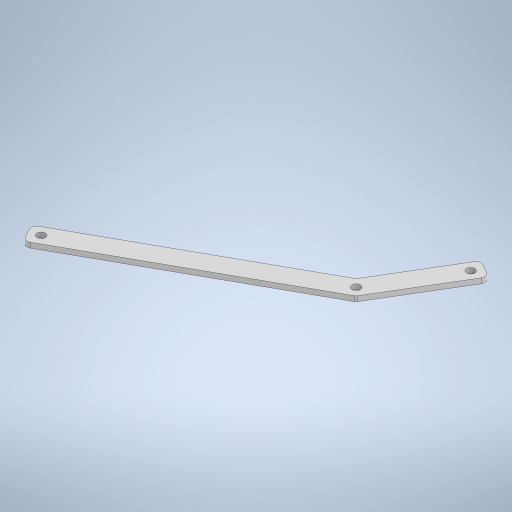
# Autodesk Inventor part: Outer Gripper Bar
Saved by Autodesk Inventor 2023 (Build 270158000, 158)
## iProperties
Created: 2023-03-01
Part Number: Outer Gripper Bar
Material: Generic
Document SubType Name: Modeling
Designer: Gabriel - T3 CAD
Density: 1 g/cm^3
Appearance: Default
Author: Gabriel - T3 CAD
Autodesk Inventor part; units mm, degrees
ref_plane "YZ Plane" through (0, 0, 0) normal (1, 0, 0) x (0, 1, 0)
ref_plane "XZ Plane" through (0, 0, 0) normal (0, 1, 0) x (-1, 0, 0)
ref_plane "XY Plane" through (0, 0, 0) normal (0, 0, 1) x (1, 0, 0)
sketch "Sketch1" plane through (0, 0, 0) normal (0, 1, 0) x (-1, 0, 0)
  line L0 (0, 76.2) -> (0, -76.2)
  line L1 (270.7338, 0) -> (-270.7338, 0)
  circle A0 centre (0, 69.85) radius 2.5797
  circle A1 centre (0, 44.45) radius 2.5797
  circle A2 centre (152.4, 158.75) radius 2.5797
  line L2 (158.75, 139.7) -> (158.75, 152.4)
  line L3 (158.75, 152.4) -> (273.05, 152.4)
  line L4 (273.05, 152.4) -> (273.05, 139.7)
  line L5 (273.05, 139.7) -> (158.75, 139.7)
  line L6 (146.05, 155.575) -> (158.75, 155.575)
  line L7 (158.75, 155.575) -> (158.75, 190.5)
  line L8 (158.75, 190.5) -> (146.05, 190.5)
  line L9 (146.05, 190.5) -> (146.05, 155.575)
  line L10 (158.75, 152.4) -> (273.05, 152.4)
  line L11 (273.05, 152.4) -> (273.05, 155.575)
  line L12 (273.05, 155.575) -> (158.75, 155.575)
  line L13 (158.75, 155.575) -> (158.75, 152.4)
  line L14 (158.75, 190.5) -> (273.05, 155.575)
  line L15 (266.7, 157.5153) -> (266.7, 155.575)
  circle A3 centre (152.4, 184.15) radius 2.5797
  circle A4 centre (152.4, 158.75) radius 2.5797
  line L16 (158.75, 155.575) -> (146.05, 155.575)
  line L17 (146.05, 155.575) -> (146.05, 152.4)
  line L18 (146.05, 152.4) -> (158.75, 152.4)
  line L19 (158.75, 152.4) -> (158.75, 155.575)
  line L20 (1.5875, 76.2) -> (-4.7625, 76.2)
  line L21 (-4.7625, 76.2) -> (-4.7625, -76.2)
  line L22 (-4.7625, -76.2) -> (1.5875, -76.2)
  line L23 (4.7625, -73.025) -> (4.7625, -41.275)
  line L24 (1.5875, -76.2) -> (1.5875, 76.2)
  line L25 (-1.5875, -76.2) -> (-1.5875, 76.2)
  circle A5 centre (0, -44.45) radius 2.5797
  circle A6 centre (0, -69.85) radius 2.5797
  line L26 (-4.7625, -38.1) -> (1.5875, -38.1)
  arc A7 (4.7625, -41.275) -> (1.5875, -38.1) centre (1.5875, -41.275) ccw
  arc A8 (1.5875, -76.2) -> (4.7625, -73.025) centre (1.5875, -73.025) ccw
  line L27 (-4.7625, 76.2) -> (4.7625, 76.2)
  line L28 (4.7625, 73.025) -> (4.7625, 41.275)
  line L29 (1.5875, 38.1) -> (-4.7625, 38.1)
  line L30 (-4.7625, 38.1) -> (-4.7625, 76.2)
  circle A9 centre (0, 69.85) radius 2.5797
  circle A10 centre (0, 44.45) radius 2.5797
  arc A11 (4.7625, 73.025) -> (1.5875, 76.2) centre (1.5875, 73.025) ccw
  arc A12 (1.5875, 38.1) -> (4.7625, 41.275) centre (1.5875, 41.275) ccw
  line L31 (152.4, 158.75) -> (27.7437, 90.2444)
  line L32 (27.7437, 90.2444) -> (0, 44.45)
  line L33 (5.4311, 41.1597) -> (-5.4311, 47.7403)
  line L34 (-5.4311, 47.7403) -> (22.7534, 94.2623)
  line L35 (32.6024, 100.1603) -> (38.8737, 96.361)
  line L36 (31.8523, 84.7712) -> (5.4311, 41.1597)
  line L37 (149.3417, 164.315) -> (155.4583, 153.185)
  line L38 (155.4583, 153.185) -> (33.0387, 85.9086)
  line L39 (21.1631, 79.3823) -> (17.6317, 85.8082)
  line L40 (23.9398, 95.3997) -> (149.3417, 164.315)
  arc A13 (23.9398, 95.3997) -> (22.7534, 94.2623) centre (25.4689, 92.6172) ccw
  arc A14 (33.0387, 85.9086) -> (31.8523, 84.7712) centre (34.5678, 83.1261) ccw
  circle A15 centre (152.4, 158.75) radius 2.5797
  circle A16 centre (0, 44.45) radius 2.5797
  line L41 (-5.4311, 47.7403) -> (5.4311, 41.1597)
  line L42 (5.4311, 41.1597) -> (3.7859, 38.4442)
  line L43 (-0.5748, 37.3738) -> (-6.0058, 40.6641)
  line L44 (-7.0762, 45.0248) -> (-5.4311, 47.7403)
  arc A17 (-7.0762, 45.0248) -> (-6.0058, 40.6641) centre (-4.3607, 43.3796) ccw
  arc A18 (-0.5748, 37.3738) -> (3.7859, 38.4442) centre (1.0704, 40.0893) ccw
  line L45 (149.3417, 164.315) -> (155.4583, 153.185)
  line L46 (155.4583, 153.185) -> (158.2408, 154.7141)
  line L47 (159.4942, 159.0258) -> (156.4359, 164.5908)
  line L48 (152.1242, 165.8442) -> (149.3417, 164.315)
  arc A19 (156.4359, 164.5908) -> (152.1242, 165.8442) centre (153.6534, 163.0616) ccw
  arc A20 (158.2408, 154.7141) -> (159.4942, 159.0258) centre (156.7116, 157.4966) ccw
  line L49 (152.4, 184.15) -> (26.6539, 114.3)
  line L50 (26.6539, 114.3) -> (0, 69.85)
  line L51 (5.4459, 66.5844) -> (-5.4459, 73.1156)
  line L52 (-5.4459, 73.1156) -> (21.6455, 118.2952)
  line L53 (31.4676, 124.2379) -> (37.756, 120.4671)
  line L54 (30.7873, 108.8455) -> (5.4459, 66.5844)
  line L55 (149.3165, 189.7011) -> (155.4835, 178.5989)
  line L56 (155.4835, 178.5989) -> (31.9686, 109.9883)
  line L57 (20.1227, 103.4081) -> (16.5622, 109.8179)
  line L58 (22.8267, 119.438) -> (149.3165, 189.7011)
  arc A21 (22.8267, 119.438) -> (21.6455, 118.2952) centre (24.3684, 116.6624) ccw
  arc A22 (31.9686, 109.9883) -> (30.7873, 108.8455) centre (33.5103, 107.2127) ccw
  circle A23 centre (152.4, 184.15) radius 2.5797
  circle A24 centre (26.6539, 114.3) radius 2.5797
  circle A25 centre (0, 69.85) radius 2.5797
  line L59 (-5.4459, 73.1156) -> (5.4459, 66.5844)
  line L60 (5.4459, 66.5844) -> (3.8132, 63.8614)
  line L61 (-0.5426, 62.7713) -> (-5.9886, 66.0368)
  line L62 (-7.0787, 70.3926) -> (-5.4459, 73.1156)
  arc A26 (-7.0787, 70.3926) -> (-5.9886, 66.0368) centre (-4.3558, 68.7598) ccw
  arc A27 (-0.5426, 62.7713) -> (3.8132, 63.8614) centre (1.0902, 65.4942) ccw
  line L63 (149.3165, 189.7011) -> (155.4835, 178.5989)
  line L64 (155.4835, 178.5989) -> (158.2591, 180.1407)
  line L65 (159.4928, 184.458) -> (156.4093, 190.0091)
  line L66 (152.092, 191.2428) -> (149.3165, 189.7011)
  arc A28 (156.4093, 190.0091) -> (152.092, 191.2428) centre (153.6338, 188.4673) ccw
  arc A29 (158.2591, 180.1407) -> (159.4928, 184.458) centre (156.7173, 182.9162) ccw
  line L67 (33.0039, 28.575) -> (33.0039, -28.575)
  line L68 (29.8289, -31.75) -> (23.4789, -31.75)
  line L69 (20.3039, -28.575) -> (20.3039, 28.575)
  line L70 (23.4789, 31.75) -> (29.8289, 31.75)
  line L71 (33.0039, 117.475) -> (33.0039, 22.225)
  line L72 (29.8289, 19.05) -> (23.4789, 19.05)
  line L73 (20.3039, 22.225) -> (20.3039, 117.475)
  line L74 (23.4789, 120.65) -> (29.8289, 120.65)
  circle A30 centre (26.6539, 25.4) radius 2.6206
  circle A31 centre (26.6539, -25.4) radius 2.6206
  circle A32 centre (26.6539, 25.4) radius 2.6206
  circle A33 centre (26.6539, 114.3) radius 2.6206
  arc A34 (33.0039, 28.575) -> (29.8289, 31.75) centre (29.8289, 28.575) ccw
  arc A35 (23.4789, 31.75) -> (20.3039, 28.575) centre (23.4789, 28.575) ccw
  arc A36 (20.3039, -28.575) -> (23.4789, -31.75) centre (23.4789, -28.575) ccw
  arc A37 (29.8289, -31.75) -> (33.0039, -28.575) centre (29.8289, -28.575) ccw
  arc A38 (20.3039, 22.225) -> (23.4789, 19.05) centre (23.4789, 22.225) ccw
  arc A39 (29.8289, 19.05) -> (33.0039, 22.225) centre (29.8289, 22.225) ccw
  arc A40 (33.0039, 117.475) -> (29.8289, 120.65) centre (29.8289, 117.475) ccw
  arc A41 (23.4789, 120.65) -> (20.3039, 117.475) centre (23.4789, 117.475) ccw
  point P0 (0, 0)
  point P1 (0, 0)
  point P2 (0, 44.45)
  point P3 (46.8631, 0)
  point P4 (2.1408, 35.7286)
  point P5 (161.0233, 156.2433)
  point P6 (2.1804, 61.1385)
  point P7 (161.0346, 181.6825)
  point P8 (33.0039, 31.75)
  point P9 (33.0039, -31.75)
  point P10 (33.0039, 120.65)
  point P11 (33.0039, 19.05)
  point P12 (20.3039, 19.05)
  point P13 (33.0039, 0)
  dimension "d4" = 5.1594
  dimension "d11" = 5.1594
  dimension "d17" = 152.4
  dimension "d56" = 12.7
  dimension "d57" = 114.3
  dimension "d58" = 3.175
  dimension "d61" = 6.35
  dimension "d63" = 5.1594
  dimension "d65" = 6.35
  dimension "d66" = 6.35
  dimension "d67" = 6.35
  dimension "d68" = 6.35
  dimension "d69" = 9.525
  dimension "d70" = 152.4
  dimension "d71" = 3.175
  dimension "d72" = 3.175
  dimension "d73" = 25.4
  dimension "d74" = 6.35
  dimension "d75" = 4.7625
  dimension "d76" = 4.7625
  dimension "d77" = 6.35
  dimension "d78" = 3.175
  dimension "d79" = 5.1594
  dimension "d80" = 25.4
  dimension "d81" = 6.35
  dimension "d82" = 4.7625
  dimension "d83" = 4.7625
  dimension "d84" = 6.35
  dimension "d85" = 3.175
  dimension "d89" = 190.5
  dimension "d92" = 150
  dimension "d94" = 142.24
  dimension "d95" = 12.7
  dimension "d96" = 3.175
  dimension "d97" = 6.35
  dimension "d98" = 3.175
  dimension "d99" = 6.35
  dimension "d100" = 3.175
  dimension "d101" = 5.1594
  dimension "d102" = 190.5
  dimension "d103" = 150
  dimension "d105" = 12.7
  dimension "d106" = 3.175
  dimension "d107" = 6.35
  dimension "d108" = 3.175
  dimension "d109" = 6.35
  dimension "d110" = 3.175
  dimension "d111" = 5.1594
  dimension "d112" = 12.7
  dimension "d113" = 12.7
  dimension "d114" = 76.2
  dimension "d115" = 4.7625
  dimension "d116" = 265.9713
  dimension "d117" = 42.1006
  dimension "d118" = 139.7
  dimension "d119" = 88.9
  dimension "d120" = 25.4
  dimension "d121" = 12.7
  dimension "d123" = 12.7
  dimension "d124" = 5.2413
  dimension "d125" = 6.35
  dimension "d126" = 6.35
  dimension "d127" = 6.35
  dimension "d128" = 6.35
  constraints: 150 end point, 49 tangent, 48 point on circle, 42 centre point, 42 point on line, 38 parallel, 24 equal radius, 18 perpendicular, 13 midpoint, 12 coincident, 5 vertical, 4 collinear, 1 concentric, 1 horizontal
  measures "d4" diameter of A0
  measures "d11" diameter of A1
  measures "d17" distance of L0.start L0.end
  measures "d56" distance of L2.start L2.end
  measures "d57" distance of L4.end L2.start
  measures "d58" distance of L11.end L3.end
  measures "d61" distance of L15.end L11.end
  measures "d63" diameter of A4
  measures "d65" distance from line of L9 A4.centre
  measures "d66" distance from line of L9 A3.centre
  measures "d67" distance from line of L8 A3.centre
  measures "d68" distance from line of L18 A4.centre
  measures "d69" distance of L27.end L20.end
  measures "d70" distance of L20.end L21.end
  measures "d71" distance between parallel lines of L23 L24
  measures "d72" distance between parallel lines of L21 L25
  measures "d73" distance of A6.centre A5.centre
  measures "d74" distance from line of L22 A6.centre
  measures "d75" distance from line of L21 A6.centre
  measures "d76" distance from line of L21 A5.centre
  measures "d77" distance from line of A5.centre L26
  measures "d78" radius of A7
  measures "d79" diameter of A6
  measures "d80" distance of A10.centre A9.centre
  measures "d81" distance from line of L20 A9.centre
  measures "d82" distance from line of L21 A9.centre
  measures "d83" distance from line of L21 A10.centre
  measures "d84" distance from line of L29 A10.centre
  measures "d85" radius of A11
  measures "d89" distance of L31.start L32.end
  measures "d92" angle of L31 L32
  measures "d94" distance of L31.start L31.end
  measures "d95" distance of L33.start L33.end
  measures "d96" radius of A13
  measures "d97" distance of L33.start point (2.141, 35.729)
  measures "d98" radius of A17
  measures "d99" distance of point (161.023, 156.243) L37.end
  measures "d100" radius of A19
  measures "d101" diameter of A15
  measures "d102" distance of L49.start L50.end
  measures "d103" angle of L49 L50
  measures "d105" distance of L54.end L52.start
  measures "d106" radius of A21
  measures "d107" distance of L54.end point (2.18, 61.138)
  measures "d108" radius of A26
  measures "d109" distance of point (161.035, 181.682) L64.start
  measures "d110" radius of A28
  measures "d111" diameter of A23
  measures "d112" distance between parallel lines of L38 L40
  measures "d113" distance between parallel lines of L56 L58
  measures "d114" diameter of L26 L1
  measures "d115" distance between parallel lines of L0 L23
  measures "d116" distance from line of L1.start L23
  measures "d117" distance from line of point (46.863, 0) L23
  measures "d118" diameter of point (0, 69.85) L1
  measures "d119" diameter of point (0, 44.45) L1
  measures "d120" distance of A4.centre A3.centre
  measures "d121" distance of L7.end L8.end
  measures "d123" distance of point (33.004, 19.05) point (20.304, 19.05)
  measures "d124" diameter of A31
  measures "d125" distance from line of L69 A31.centre
  measures "d126" distance from line of L69 A30.centre
  measures "d127" distance from line of L73 A32.centre
  measures "d128" distance from line of L73 A33.centre
sketch "Sketch2" plane through (0, 0, 0) normal (1, 0, 0) x (0, 1, 0)
  line L0 (0, 76.2) -> (0, -76.2)
  line L1 (270.7338, 0) -> (-270.7338, 0)
  circle A0 centre (0, 69.85) radius 2.5797
  circle A1 centre (0, 44.45) radius 2.5797
  circle A2 centre (188.7991, 19.05) radius 2.5797
  line L2 (195.1491, 0) -> (195.1491, 12.7)
  line L3 (195.1491, 12.7) -> (309.4491, 12.7)
  line L4 (309.4491, 12.7) -> (309.4491, 0)
  line L5 (309.4491, 0) -> (195.1491, 0)
  line L6 (182.4491, 15.875) -> (195.1491, 15.875)
  line L7 (195.1491, 15.875) -> (195.1491, 50.8)
  line L8 (195.1491, 50.8) -> (182.4491, 50.8)
  line L9 (182.4491, 50.8) -> (182.4491, 15.875)
  line L10 (195.1491, 12.7) -> (309.4491, 12.7)
  line L11 (309.4491, 12.7) -> (309.4491, 15.875)
  line L12 (309.4491, 15.875) -> (195.1491, 15.875)
  line L13 (195.1491, 15.875) -> (195.1491, 12.7)
  line L14 (195.1491, 50.8) -> (309.4491, 15.875)
  line L15 (303.0991, 17.8153) -> (303.0991, 15.875)
  circle A3 centre (188.7991, 44.45) radius 2.5797
  circle A4 centre (188.7991, 19.05) radius 2.5797
  line L16 (195.1491, 15.875) -> (182.4491, 15.875)
  line L17 (182.4491, 15.875) -> (182.4491, 12.7)
  line L18 (182.4491, 12.7) -> (195.1491, 12.7)
  line L19 (195.1491, 12.7) -> (195.1491, 15.875)
  line L20 (1.5875, 76.2) -> (-4.7625, 76.2)
  line L21 (-4.7625, 76.2) -> (-4.7625, -76.2)
  line L22 (-4.7625, -76.2) -> (1.5875, -76.2)
  line L23 (4.7625, -73.025) -> (4.7625, -41.275)
  line L24 (1.5875, -76.2) -> (1.5875, 76.2)
  line L25 (-1.5875, -76.2) -> (-1.5875, 76.2)
  circle A5 centre (0, -44.45) radius 2.5797
  circle A6 centre (0, -69.85) radius 2.5797
  line L26 (-4.7625, -38.1) -> (1.5875, -38.1)
  arc A7 (4.7625, -41.275) -> (1.5875, -38.1) centre (1.5875, -41.275) ccw
  arc A8 (1.5875, -76.2) -> (4.7625, -73.025) centre (1.5875, -73.025) ccw
  line L27 (-4.7625, 76.2) -> (4.7625, 76.2)
  line L28 (4.7625, 73.025) -> (4.7625, 41.275)
  line L29 (1.5875, 38.1) -> (-4.7625, 38.1)
  line L30 (-4.7625, 38.1) -> (-4.7625, 76.2)
  circle A9 centre (0, 69.85) radius 2.5797
  circle A10 centre (0, 44.45) radius 2.5797
  arc A11 (4.7625, 73.025) -> (1.5875, 76.2) centre (1.5875, 73.025) ccw
  arc A12 (1.5875, 38.1) -> (4.7625, 41.275) centre (1.5875, 41.275) ccw
  line L31 (188.7991, 19.05) -> (51.8933, 57.638)
  line L32 (51.8933, 57.638) -> (0, 44.45)
  line L33 (1.564, 38.2956) -> (-1.564, 50.6044)
  line L34 (-1.564, 50.6044) -> (51.1538, 64.0019)
  line L35 (62.311, 61.2991) -> (64.117, 54.1926)
  line L36 (50.9838, 50.855) -> (1.564, 38.2956)
  line L37 (190.5218, 25.1619) -> (187.0764, 12.9381)
  line L38 (187.0764, 12.9381) -> (52.6271, 50.8337)
  line L39 (39.5846, 54.5099) -> (41.5738, 61.5673)
  line L40 (52.7972, 63.9806) -> (190.5218, 25.1619)
  arc A13 (52.7972, 63.9806) -> (51.1538, 64.0019) centre (51.9358, 60.9247) ccw
  arc A14 (52.6271, 50.8337) -> (50.9838, 50.855) centre (51.7658, 47.7778) ccw
  circle A15 centre (188.7991, 19.05) radius 2.5797
  circle A16 centre (0, 44.45) radius 2.5797
  line L41 (-1.564, 50.6044) -> (1.564, 38.2956)
  line L42 (1.564, 38.2956) -> (-1.5131, 37.5136)
  line L43 (-5.3723, 39.8088) -> (-6.9364, 45.9631)
  line L44 (-4.6412, 49.8223) -> (-1.564, 50.6044)
  arc A17 (-4.6412, 49.8223) -> (-6.9364, 45.9631) centre (-3.8592, 46.7452) ccw
  arc A18 (-5.3723, 39.8088) -> (-1.5131, 37.5136) centre (-2.2952, 40.5908) ccw
  line L45 (190.5218, 25.1619) -> (187.0764, 12.9381)
  line L46 (187.0764, 12.9381) -> (190.1323, 12.0768)
  line L47 (194.0496, 14.2714) -> (195.7723, 20.3833)
  line L48 (193.5777, 24.3005) -> (190.5218, 25.1619)
  arc A19 (195.7723, 20.3833) -> (193.5777, 24.3005) centre (192.7163, 21.2446) ccw
  arc A20 (190.1323, 12.0768) -> (194.0496, 14.2714) centre (190.9937, 15.1327) ccw
  line L49 (194.0712, 39.6953) -> (195.7661, 45.8149)
  arc A21 (190.164, 37.4829) -> (194.0712, 39.6953) centre (191.0114, 40.5427) ccw
  arc A22 (195.7661, 45.8149) -> (193.5538, 49.7222) centre (192.7063, 46.6624) ccw
  line L50 (187.1042, 38.3304) -> (190.164, 37.4829)
  line L51 (193.5538, 49.7222) -> (190.494, 50.5696)
  circle A23 centre (188.7991, 44.45) radius 2.5797
  line L52 (190.494, 50.5696) -> (187.1042, 38.3304)
  line L53 (190.494, 50.5696) -> (187.1042, 38.3304)
  line L54 (60.5746, 86.5522) -> (62.4129, 79.4541)
  line L55 (187.1042, 38.3304) -> (50.9384, 76.043)
  line L56 (188.7991, 44.45) -> (50.1736, 82.8439)
  line L57 (51.0487, 89.1906) -> (190.494, 50.5696)
  line L58 (49.2949, 76.0568) -> (1.592, 63.7028)
  line L59 (-1.592, 75.9972) -> (49.4052, 89.2043)
  line L60 (50.1736, 82.8439) -> (0, 69.85)
  arc A24 (50.9384, 76.043) -> (49.2949, 76.0568) centre (50.0909, 72.9832) ccw
  arc A25 (51.0487, 89.1906) -> (49.4052, 89.2043) centre (50.2012, 86.1307) ccw
  circle A26 centre (50.1736, 82.8439) radius 2.5797
  line L61 (37.8792, 79.6599) -> (39.8363, 86.7262)
  line L62 (1.592, 63.7028) -> (-1.592, 75.9972)
  line L63 (1.592, 63.7028) -> (-1.4816, 62.9068)
  line L64 (-1.592, 75.9972) -> (1.592, 63.7028)
  circle A27 centre (0, 69.85) radius 2.5797
  line L65 (-4.6656, 75.2012) -> (-1.592, 75.9972)
  arc A28 (-5.3512, 65.1844) -> (-1.4816, 62.9068) centre (-2.2776, 65.9804) ccw
  line L66 (-5.3512, 65.1844) -> (-6.9432, 71.3316)
  arc A29 (-4.6656, 75.2012) -> (-6.9432, 71.3316) centre (-3.8696, 72.1276) ccw
  line L67 (124.3721, 28.575) -> (124.3721, -28.575)
  line L68 (121.1971, -31.75) -> (114.8471, -31.75)
  line L69 (111.6721, -28.575) -> (111.6721, 28.575)
  line L70 (114.8471, 31.75) -> (121.1971, 31.75)
  line L71 (51.8536, 89.7417) -> (124.5484, 28.1948)
  line L72 (124.92, 23.72) -> (120.8168, 18.8737)
  line L73 (116.3421, 18.5021) -> (43.6473, 80.0491)
  line L74 (43.2757, 84.5238) -> (47.3789, 89.3701)
  circle A30 centre (118.0221, 25.4) radius 2.6206
  circle A31 centre (118.0221, -25.4) radius 2.6206
  circle A32 centre (118.0221, 25.4) radius 2.6206
  circle A33 centre (50.1736, 82.8439) radius 2.6206
  arc A34 (124.3721, 28.575) -> (121.1971, 31.75) centre (121.1971, 28.575) ccw
  arc A35 (114.8471, 31.75) -> (111.6721, 28.575) centre (114.8471, 28.575) ccw
  arc A36 (111.6721, -28.575) -> (114.8471, -31.75) centre (114.8471, -28.575) ccw
  arc A37 (121.1971, -31.75) -> (124.3721, -28.575) centre (121.1971, -28.575) ccw
  arc A38 (116.3421, 18.5021) -> (120.8168, 18.8737) centre (118.3937, 20.9253) ccw
  arc A39 (124.92, 23.72) -> (124.5484, 28.1948) centre (122.4968, 25.7716) ccw
  arc A40 (51.8536, 89.7417) -> (47.3789, 89.3701) centre (49.802, 87.3186) ccw
  arc A41 (43.2757, 84.5238) -> (43.6473, 80.0491) centre (45.6989, 82.4723) ccw
  line L75 (50.1736, 82.8439) -> (118.0221, 25.4)
  line L76 (118.0221, -25.4) -> (118.0221, 25.4)
  line L77 (127.9831, -605.0736) -> (127.9831, -452.6736)
  line L78 (178.1568, -446.0297) -> (246.0052, -503.4736)
  line L79 (246.0052, -503.4736) -> (246.0052, -554.2736)
  line L80 (78.5716, -330.2354) -> (78.5716, -190.5354)
  line L81 (78.5716, -190.5354) -> (172.9711, -203.2354)
  line L82 (172.9711, -203.2354) -> (256.0081, -234.9854)
  line L83 (256.0081, -234.9854) -> (256.0081, -285.7854)
  line L84 (78.5716, -260.3854) -> (256.0081, -260.3854)
  line L85 (127.9831, -528.8736) -> (246.0052, -528.8736)
  line L86 (127.9831, -459.0236) -> (178.1568, -446.0297)
  line L87 (78.5716, -190.5354) -> (267.3706, -215.9354)
  line L88 (267.3706, -215.9354) -> (267.3706, -260.3854)
  point P0 (0, 0)
  point P1 (0, 0)
  point P2 (0, 44.45)
  point P3 (46.8631, 0)
  point P4 (-4.5903, 36.7316)
  point P5 (193.1883, 11.2155)
  point P6 (193.2238, 36.6355)
  point P7 (-4.5552, 62.1108)
  point P8 (124.3721, 31.75)
  point P9 (124.3721, -31.75)
  point P10 (49.4304, 91.7933)
  point P11 (126.9715, 26.1432)
  point P12 (118.7653, 16.4505)
  point P13 (124.3721, 0)
  point P14 (118.0221, 0)
  dimension "d145" = 5.1594
  dimension "d146" = 5.1594
  dimension "d147" = 152.4
  dimension "d148" = 12.7
  dimension "d149" = 114.3
  dimension "d150" = 3.175
  dimension "d151" = 6.35
  dimension "d152" = 5.1594
  dimension "d153" = 6.35
  dimension "d154" = 6.35
  dimension "d155" = 6.35
  dimension "d156" = 6.35
  dimension "d157" = 9.525
  dimension "d158" = 152.4
  dimension "d159" = 3.175
  dimension "d160" = 3.175
  dimension "d161" = 25.4
  dimension "d162" = 6.35
  dimension "d163" = 4.7625
  dimension "d164" = 4.7625
  dimension "d165" = 6.35
  dimension "d166" = 3.175
  dimension "d167" = 5.1594
  dimension "d168" = 25.4
  dimension "d169" = 6.35
  dimension "d170" = 4.7625
  dimension "d171" = 4.7625
  dimension "d172" = 6.35
  dimension "d173" = 3.175
  dimension "d174" = 190.5
  dimension "d175" = 150
  dimension "d176" = 142.24
  dimension "d177" = 12.7
  dimension "d178" = 3.175
  dimension "d179" = 6.35
  dimension "d180" = 3.175
  dimension "d181" = 6.35
  dimension "d182" = 3.175
  dimension "d183" = 5.1594
  dimension "d184" = 190.5
  dimension "d185" = 150
  dimension "d186" = 12.7
  dimension "d187" = 3.175
  dimension "d188" = 6.35
  dimension "d189" = 3.175
  dimension "d190" = 6.35
  dimension "d191" = 3.175
  dimension "d192" = 5.1594
  dimension "d193" = 12.7
  dimension "d194" = 12.7
  dimension "d195" = 76.2
  dimension "d196" = 4.7625
  dimension "d197" = 265.9713
  dimension "d198" = 42.1006
  dimension "d199" = 139.7
  dimension "d200" = 88.9
  dimension "d201" = 25.4
  dimension "d202" = 12.7
  dimension "d203" = 12.7
  dimension "d204" = 5.2413
  dimension "d205" = 6.35
  dimension "d206" = 6.35
  dimension "d207" = 6.35
  dimension "d208" = 6.35
  constraints: 182 end point, 49 tangent, 48 point on circle, 44 point on line, 42 centre point, 38 parallel, 24 equal radius, 19 midpoint, 18 perpendicular, 12 coincident, 8 vertical, 5 collinear, 3 horizontal, 2 equal length, 1 concentric
  measures "d145" diameter of A0
  measures "d146" diameter of A1
  measures "d147" distance of L0.start L0.end
  measures "d148" distance of L2.start L2.end
  measures "d149" distance of L4.end L2.start
  measures "d150" distance of L11.end L3.end
  measures "d151" distance of L15.end L11.end
  measures "d152" diameter of A4
  measures "d153" distance from line of L9 A4.centre
  measures "d154" distance from line of L9 A3.centre
  measures "d155" distance from line of L8 A3.centre
  measures "d156" distance from line of L18 A4.centre
  measures "d157" distance of L27.end L20.end
  measures "d158" distance of L20.end L21.end
  measures "d159" distance between parallel lines of L23 L24
  measures "d160" distance between parallel lines of L21 L25
  measures "d161" distance of A6.centre A5.centre
  measures "d162" distance from line of L22 A6.centre
  measures "d163" distance from line of L21 A6.centre
  measures "d164" distance from line of L21 A5.centre
  measures "d165" distance from line of A5.centre L26
  measures "d166" radius of A7
  measures "d167" diameter of A6
  measures "d168" distance of A10.centre A9.centre
  measures "d169" distance from line of L20 A9.centre
  measures "d170" distance from line of L21 A9.centre
  measures "d171" distance from line of L21 A10.centre
  measures "d172" distance from line of L29 A10.centre
  measures "d173" radius of A11
  measures "d174" distance of L31.start L32.end
  measures "d175" angle of L31 L32
  measures "d176" distance of L31.start L31.end
  measures "d177" distance of L33.start L33.end
  measures "d178" radius of A13
  measures "d179" distance of L33.start point (-4.59, 36.732)
  measures "d180" radius of A17
  measures "d181" distance of point (193.188, 11.215) L37.end
  measures "d182" radius of A19
  measures "d183" diameter of A15
  measures "d184" distance of L56.start L60.end
  measures "d185" angle of L56 L60
  measures "d186" distance of L58.end L59.start
  measures "d187" radius of A25
  measures "d188" distance of L58.end point (-4.555, 62.111)
  measures "d189" radius of A29
  measures "d190" distance of point (193.224, 36.635) L50.start
  measures "d191" radius of A22
  measures "d192" diameter of A23
  measures "d193" distance between parallel lines of L38 L40
  measures "d194" distance between parallel lines of L55 L57
  measures "d195" diameter of L26 L1
  measures "d196" distance between parallel lines of L0 L23
  measures "d197" distance from line of L1.start L23
  measures "d198" distance from line of point (46.863, 0) L23
  measures "d199" diameter of point (0, 69.85) L1
  measures "d200" diameter of point (0, 44.45) L1
  measures "d201" distance of A4.centre A3.centre
  measures "d202" distance of L7.end L8.end
  measures "d203" distance of point (126.972, 26.143) point (118.765, 16.451)
  measures "d204" diameter of A31
  measures "d205" distance from line of L69 L76.start
  measures "d206" distance from line of L69 A30.centre
  measures "d207" distance from line of L73 L75.end
  measures "d208" distance from line of L73 L75.start
extrude "Extrusion1" add sketch "Sketch1" along normal blind 3.175 contours L20 L24 L50 A0 L0 | L20 L52 L57 L50 L27 | L0 A0 L25 L20 | A11 L50 L24 | L27 L50 A11 | L25 A0 L51 L21 L52 L20 | L50 L24 A0 | L50 A11 L28 L51 A0 L24 | L50 L73 L54 L51 L28 A11 | A0 L24 A27 L0 | L0 A27 L61 L25 A0 | A0 L25 L61 L21 L51 | L57 L52 L73 L50 | L21 L51 L52 | A0 L51 L28 L60 A27 L24 | L21 L61 A26 L62 L51 | L73 L52 A21 L58 L74 A40 L49 A33 L50 | L50 A33 L49 A40 L71 L56 A22 L54 L73 | L51 L60 L28 | A40 L74 L58 L53 L49 | L49 L9 L56 L71 A40 | L53 L58 L9 L49 | L49 A3 L55 L56 L9 | L9 L58 L55 A3 L49 | L55 A3 L66 L8 A28 L65 L7 A29 L64 | L66 A28 L8 | L7 L65 A29
body "Solid1"
